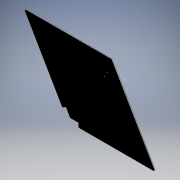
# Autodesk Inventor part: Acrylic_top
Saved by Autodesk Inventor 2019.4 (Build 234330000, 330)
## iProperties
Created: 2020-02-04
Part Number: Acrylic_top
Material: Generic
Document SubType Name: Modeling
Designer: Jorian Brusind
Density: 1 g/cm^3
Appearance: Default
Author: Jorian Brusind
Autodesk Inventor part; units mm, degrees
ref_plane "YZ Plane" through (0, 0, 0) normal (1, 0, 0) x (0, 1, 0)
ref_plane "XZ Plane" through (0, 0, 0) normal (0, 1, 0) x (-1, 0, 0)
ref_plane "XY Plane" through (0, 0, 0) normal (0, 0, 1) x (1, 0, 0)
sketch "Sketch7" plane through (0, 0, 0) normal (0, 0, 1) x (1, 0, 0)
  line L0 (182.5, 316.0993) -> (365, 0)
  line L1 (365, 0) -> (182.5, -316.0993)
  line L2 (182.5, -316.0993) -> (-182.5, -316.0993)
  line L3 (-182.5, -316.0993) -> (-365, 0)
  line L4 (-365, 0) -> (-182.5, 316.0993)
  line L5 (-182.5, 316.0993) -> (182.5, 316.0993)
  line L6 (0, 0) -> (-182.5, 316.0993)
  line L7 (0, 0) -> (365, 0)
  line L8 (0, 0) -> (0, 100)
  line L9 (0, 0) -> (100, 0) construction
  dimension "d56" = 365
  dimension "d69" = 100
  dimension "d70" = 90
  dimension "d71" = 30
  constraints: 20 end point, 1 coincident, 1 horizontal, 1 perpendicular, 1 vertical, 13 other
  measures "d56" distance of L4.end L0.start
  measures "d69" distance of L6.start L8.end
  measures "d70" angle of L9 L8
  measures "d71" angle of L8 L6
extrude "Extrusion6" add sketch "Sketch7" along normal blind 3 contours L0 L7 L6 L5
sketch "Sketch8" plane through (0, 0, 3) normal (0, 0, 1) x (1, 0, 0)
  line L0 (37.6554, -30.2211) -> (-7.3446, 47.7211)
  line L1 (-7.3446, 47.7211) -> (-37.6554, 30.2211)
  line L2 (-37.6554, 30.2211) -> (7.3446, -47.7211)
  line L3 (7.3446, -47.7211) -> (37.6554, -30.2211)
  line L4 (37.6554, -30.2211) -> (-37.6554, 30.2211) construction
  line L5 (-7.3446, 47.7211) -> (7.3446, -47.7211) construction
  line L6 (37.6554, -30.2211) -> (127.6554, -30.2211) construction
  line L7 (-45, 17.5) -> (45, 17.5)
  line L8 (45, 17.5) -> (45, -17.5)
  line L9 (45, -17.5) -> (-45, -17.5)
  line L10 (-45, -17.5) -> (-45, 17.5)
  line L11 (-182.5, 316.0993) -> (0, 0) projected
  line L12 (-45, 17.5) -> (45, -17.5) construction
  line L13 (45, 17.5) -> (-45, -17.5) construction
  line L14 (-45, 17.5) -> (45, 17.5) construction
  dimension "d60" = 90
  dimension "d61" = 120
  dimension "d62" = 35
  dimension "d63" = 90
  dimension "d64" = 0
  dimension "d65" = 35
  constraints: 28 end point, 4 midpoint, 4 parallel, 3 horizontal, 2 equal length, 2 perpendicular
  measures "d60" distance of L0.start L0.end
  measures "d61" angle of L6 L0
  measures "d62" distance of L1.end L0.end
  measures "d63" distance of L7.start L7.end
  measures "d64" distance between parallel lines of L7 L14
  measures "d65" distance of L7.end L8.end
extrude "Extrusion7" cut sketch "Sketch8" against normal blind 3
sketch "Sketch9" plane through (0, 0, 3) normal (0, 0, 1) x (1, 0, 0)
  line L0 (0, 0) -> (152.5, 264.1377)
  line L1 (0, 0) -> (305, 0) construction
  line L2 (152.5, 264.1377) -> (163.7583, 257.6377)
  line L3 (152.5, 264.1377) -> (165.5, 264.1377) construction
  circle A0 centre (163.7583, 257.6377) radius 1.75
  line L4 (163.7583, 257.6377) -> (153.7583, 240.3172)
  circle A1 centre (153.7583, 240.3172) radius 1.75
  dimension "d72" = 305
  dimension "d73" = 60
  dimension "d74" = 13
  dimension "d75" = 30
  dimension "d76" = 3.5
  dimension "d77" = 20
  dimension "d78" = 90
  dimension "d79" = 3.5
  constraints: 10 end point, 2 centre point, 2 coincident, 2 equal length, 2 horizontal
  measures "d72" distance of L0.start L0.end
  measures "d73" angle of L1 L0
  measures "d74" distance of L0.end L2.end
  measures "d75" angle of L2 L3
  measures "d76" diameter of A0
  measures "d77" distance of L4.start L4.end
  measures "d78" angle of L2 L4
  measures "d79" diameter of A1
extrude "Extrusion8" cut sketch "Sketch9" against normal blind 3
fillet "Fillet1" radius 5 3 edges at (182.5, 316.0993, 1.5) (365, 0, 1.5) (-182.5, 316.0993, 1.5)
fillet "Fillet2" radius 2 2 edges at (45, 17.5, 1.5) (-7.3446, 47.7211, 1.5)
fillet "Fillet3" radius 2 2 edges at (45, 0, 1.5) (10.1036, 17.5, 1.5)
fillet "Fillet4" radius 2 1 edges at (-22.5, 38.9711, 1.5)
body "Solid2"
